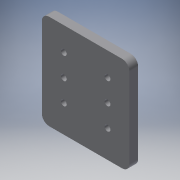
# Autodesk Inventor part: Wheel height spacers
Saved by Autodesk Inventor 2018 (Build 220112000, 112)
## iProperties
Created: 2018-05-02
Part Number: Wheel height spacers
Material: Generic
Document SubType Name: Modeling
Designer: Ajith Thomas
Density: 1 g/cm^3
Appearance: Default
Author: Ajith Thomas
Autodesk Inventor part; units mm, degrees
ref_plane "YZ Plane" through (0, 0, 0) normal (1, 0, 0) x (0, 1, 0)
ref_plane "XZ Plane" through (0, 0, 0) normal (0, 1, 0) x (-1, 0, 0)
ref_plane "XY Plane" through (0, 0, 0) normal (0, 0, 1) x (1, 0, 0)
sketch "Sketch1" plane through (0, 0, 0) normal (0, 0, 1) x (1, 0, 0)
  line L0 (0, -5.0856) -> (0, -49.3) projected
  line L1 (0, -54.8) -> (-50, -54.8) projected
  line L2 (-50, -5.0856) -> (-50, -49.3) projected
  line L3 (-5.3931, 0) -> (-44.6069, 0) projected
  line L4 (-50, -27.1928) -> (0, -27.1928) construction
  line L5 (-25, 0) -> (-25, -54.8) construction
  line L6 (-55, 5.1) -> (5, 5.1)
  line L7 (5, 5.1) -> (5, -59.9)
  line L8 (5, -59.9) -> (-55, -59.9)
  line L9 (-55, -59.9) -> (-55, 5.1)
  line L10 (-55, 5.1) -> (5, -59.9) construction
  line L11 (5, 5.1) -> (-55, -59.9) construction
  point P0 (0, 0)
  point P1 (-25, -27.4)
  dimension "d0" = 60
  dimension "d1" = 65
  constraints: 16 end point, 7 midpoint, 2 parallel, 1 horizontal, 1 perpendicular
  measures "d0" distance of L7.end L8.end
  measures "d1" distance of L6.end L7.end
extrude "Extrusion1" add sketch "Sketch1" along normal blind 6
sketch "Sketch2" plane through (0, 0, 6) normal (0, 0, 1) x (1, 0, 0)
  circle A0 centre (-40, -11) radius 2 projected
  circle A1 centre (-40, -26) radius 2 projected
  circle A2 centre (-40, -41) radius 2 projected
  circle A3 centre (-10, -41) radius 2 projected
  circle A4 centre (-10, -26) radius 2 projected
  circle A5 centre (-10, -11) radius 2 projected
  point P0 (0, 0)
extrude "Extrusion2" cut sketch "Sketch2" against normal blind 6
fillet "Fillet1" radius 5 4 edges at (-55, -59.9, 3) (-55, 5.1, 3) (5, -59.9, 3) (5, 5.1, 3)
body "Solid1"
